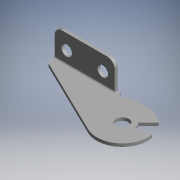
# Autodesk Inventor part: MHPUS306-Ab_free_left
Saved by Autodesk Inventor 2017.3 (Build 213256000, 256)
## iProperties
Part Number: MHPUS306-Ab_free_left
Material: Generic
Catalog Web Link: www.cadenas.de
Description: MHPUS_b_free_left-Cable Carriers Flap Open - Close Type
Vendor: MISUMI
Document SubType Name: Modeling
Designer: partserver
Manufacturer: MISUMI
Mass: 4.40445 g
Surface Area: 49.8583 cm^2
Volume: 4.40445 cm^3
Density: 1 g/cm^3
Appearance: PSOLRGB-192-192-192
Category: PARTsolutions
Company: MISUMI
Title: MHPUS306-Ab_free_left
Author: Cadenas PARTsolutions
Comments: Cable Carriers Flap Open - Close Type
PSOL_IDENT_0: {$CADENAS_DATA\23d-libs\misumi\metric\07_slide_rails\mhpus_bracket_free_left.prj},195 {VTYP=3D},{NB=
PSOL_IDENT_1: MHPUS306-Ab_free_left},{LINA=MHPUS306-Ab_free_left},{NN=MHPUS_b_free_left},{DATE=30.06.2021 12:53:59
PSOL_IDENT_2: },{GEOMDATE=28.08.2009 10:42:00},{VERSION=},{LINEID=80},{WBVAR=AD},{WBNUMERIC=}  {NB=MHPUS306-Ab_fre
PSOL_IDENT_3: e_left},{LINA=MHPUS306-Ab_free_left},{KT=DUMMY},{PN=MHPUS306-A},{NO=306},{MAT=Low Carbon Steel},{ST=
PSOL_IDENT_4: Trivalent Bright Chromate Plating},{AD=A},{ADALG= 'A', 'Outer circumference', 'B', 'Inner circumfere
PSOL_IDENT_5: nce' },{HH=34},{F=40},{T=24},{J=20},{N=7.0},{LL=60},{P1F=35.6},{P2F=55.6},{P1FX=32},{P2FX=52},{R4=8.
PSOL_IDENT_6: 000},{R1=2.000},{R2=5.000},{R24=35.000},{R25=10.000},{R26=7.500},{END=1}
NB: MHPUS306-Ab_free_left
NN: MHPUS_b_free_left
NT: Cable Carriers Flap Open - Close Type
NBSYN: $PN.b_free_left
LINA: MHPUS306-Ab_free_left
CATALOG: Misumi
PN: MHPUS306-A
NO: 306
MAT: Low Carbon Steel
ST: Trivalent Bright Chromate Plating
AD: Outer circumference
HH: 34
F: 40
T: 24
J: 20
N: 7
LL: 60
P1F: 35.6
P2F: 55.6
P1FX: 32
P2FX: 52
R4: 8
R1: 2
R2: 5
R24: 35
R25: 10
R26: 7.5
SUPPLIER: MISUMI
ARTICLENO: MHPUS306-Ab_free_left
BOMINFO: MHPUS306-Ab_free_left
CREATOR: CADENAS GmbH
Autodesk Inventor part; units mm, degrees
sketch "Sketch_10" plane through (0, 0, 0) normal (0, 0, 1) x (1, 0, 0)
  arc A0 (-16.7417, 19.952) -> (7.4171, 1.7034) centre (0, 17) ccw
  line L0 (7.4171, 1.7034) -> (58.0834, 26.2707)
  arc A1 (58.0834, 26.2707) -> (60, 29.33) centre (56.6, 29.33) ccw
  line L1 (60, 29.33) -> (60, 34)
  line L2 (60, 34) -> (0, 34)
  arc A2 (0, 34) -> (-12.0208, 29.0208) centre (0, 17) ccw
  line L3 (-12.0208, 29.0208) -> (-5.3033, 22.3033)
  arc A3 (-5.3033, 22.3033) -> (-7.3861, 18.3024) centre (0, 17) ccw
  line L4 (-7.3861, 18.3024) -> (-16.7417, 19.952)
  circle A4 centre (0, 17) radius 4.25
  constraints: 10 end point, 8 point on circle, 5 centre point
extrude "Extrusion1" add sketch "Sketch_10" against normal blind 20
sketch "Sketch_11" plane through (0, 0, 0) normal (1, 0, 0) x (0, 1, 0)
  line L0 (39, 5) -> (-5, 5)
  line L1 (-5, 5) -> (-5, -25)
  line L2 (-5, -25) -> (39, -25)
  line L3 (39, -25) -> (39, 5)
  line L4 (32, 0) -> (0, 0)
  line L5 (0, 0) -> (0, -2)
  line L6 (0, -2) -> (31, -2)
  arc A0 (32, -3) -> (31, -2) centre (31, -3) ccw
  line L7 (32, -3) -> (32, -20)
  line L8 (32, -20) -> (34, -20)
  line L9 (34, -20) -> (34, -2)
  arc A1 (34, -2) -> (32, 0) centre (32, -2) ccw
  constraints: 20 end point, 4 point on circle, 2 centre point
extrude "Extrusion2" cut sketch "Sketch_11" along normal mid plane 188
sketch "Sketch_3" plane through (0, 0, 0) normal (0, 1, 0) x (-1, 0, 0)
  line L0 (22, -25) -> (22, 5)
  line L1 (22, 5) -> (-65, 5)
  line L2 (-65, 5) -> (-65, -25)
  line L3 (-65, -25) -> (22, -25)
  line L4 (17, -2) -> (17, 0)
  line L5 (17, 0) -> (-60, 0)
  line L6 (-60, 0) -> (-60, -15)
  arc A0 (-60, -15) -> (-55, -20) centre (-55, -15) ccw
  line L7 (-55, -20) -> (-25, -20)
  arc A1 (-25, -20) -> (-20, -15) centre (-25, -15) ccw
  line L8 (-20, -15) -> (-20, -2)
  line L9 (-20, -2) -> (17, -2)
  constraints: 20 end point, 4 point on circle, 2 centre point
extrude "Extrusion3" cut sketch "Sketch_3" along normal blind 34
sketch "Sketch_1" plane through (0, 34, 0) normal (0, 1, 0) x (1, 0, 0)
  circle A0 centre (28, 10) radius 3.5
  constraints: 1 centre point
extrude "Extrusion4" cut sketch "Sketch_1" along normal mid plane 4
sketch "Sketch_2" plane through (0, 34, 0) normal (0, 1, 0) x (1, 0, 0)
  circle A0 centre (52, 10) radius 3.5
  constraints: 1 centre point
extrude "Extrusion5" cut sketch "Sketch_2" along normal mid plane 4
sketch "Sketch_7" plane through (0, 0, 0) normal (0, 0, 1) x (1, 0, 0)
  circle A0 centre (15, 34) radius 2.5
  constraints: 1 centre point
extrude "Extrusion6" cut sketch "Sketch_7" against normal blind 20
ref_plane "fix_end_l_XY" through (0, 17, 0) normal (0, 0, 1) x (1, 0, 0)
ref_plane "fix_end_l_YZ" through (0, 17, 0) normal (1, 0, 0) x (0, 1, 0)
ref_plane "fix_end_l_ZX" through (0, 17, 0) normal (0, 1, 0) x (0, 0, 1)
ref_plane "free_end_l_XY" through (0, 17, -2) normal (0, 0, 1) x (1, 0, 0)
ref_plane "free_end_l_YZ" through (0, 17, -2) normal (1, 0, 0) x (0, 1, 0)
ref_plane "free_end_l_ZX" through (0, 17, -2) normal (0, 1, 0) x (0, 0, 1)
ref_plane "l_to_r_XY" through (0, 17, -27.8) normal (0, 0, 1) x (1, 0, 0)
ref_plane "l_to_r_YZ" through (0, 17, -27.8) normal (1, 0, 0) x (0, 1, 0)
ref_plane "l_to_r_ZX" through (0, 17, -27.8) normal (0, 1, 0) x (0, 0, 1)
ref_plane "to_clip5_XY" through (0, 17, -10) normal (1, 0, 0) x (0, 0, -1)
ref_plane "to_clip5_YZ" through (0, 17, -10) normal (0, 0, -1) x (0, 1, 0)
ref_plane "to_clip5_ZX" through (0, 17, -10) normal (0, 1, 0) x (1, 0, 0)
body "Solid1"
